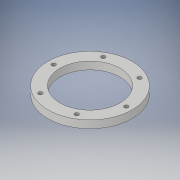
# Autodesk Inventor part: BearingRing
Saved by Autodesk Inventor 2019 (Build 230136000, 136)
## iProperties
Created: 2018-12-09
Part Number: BearingRing
Material: Generic
Document SubType Name: Modeling
Designer: steelen
Density: 1 g/cm^3
Appearance: Default
Author: steelen
Autodesk Inventor part; units mm, degrees
ref_plane "YZ Plane" through (0, 0, 0) normal (1, 0, 0) x (0, 1, 0)
ref_plane "XZ Plane" through (0, 0, 0) normal (0, 1, 0) x (-1, 0, 0)
ref_plane "XY Plane" through (0, 0, 0) normal (0, 0, 1) x (1, 0, 0)
sketch "Sketch1" plane through (0, 0, 0) normal (0, 1, 0) x (-1, 0, 0)
  circle A0 centre (0, 0) radius 50
  circle A1 centre (0, 0) radius 69.85
  dimension "d0" = 139.7
  dimension "d1" = 100
  constraints: 2 centre point, 2 coincident
  measures "d0" diameter of A1
  measures "d1" diameter of A0
extrude "Extrusion1" add sketch "Sketch1" along normal blind 12.7
sketch "Sketch2" plane through (0, 12.7, 0) normal (0, 1, 0) x (1, 0, 0)
  circle A0 centre (0, 0) radius 69.85 projected
  line L0 (-69.85, 0) -> (-60.325, 0)
  point P0 (-30.1625, 52.243)
  point P1 (30.1625, 52.243)
  point P2 (60.325, 0)
  point P3 (30.1625, -52.243)
  point P4 (-30.1625, -52.243)
  dimension "d4" = 9.525
  dimension "d7" = 360
  constraints: 2 end point, 2 horizontal, 1 horizontal alignment, 8 other
  measures "d4" distance of L0.start L0.end
hole "Hole1" at (-60.325, 12.7, 0) at (-30.1625, 12.7, -52.243) at (30.1625, 12.7, -52.243) at (60.325, 12.7, 0) at (30.1625, 12.7, 52.243) at (-30.1625, 12.7, 52.243) direction (0, -1, 0) diameter 6.5278 end through all clearance for "Socket Head Cap Screw" size "1/4" standard "Ansi Unified Screw Threads"
body "Solid1"
